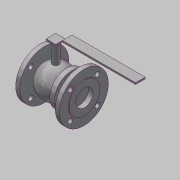
# Autodesk Inventor part: BALL VALVE FLANGED DN65
Saved by Autodesk Inventor 2017 (Build 210142000, 142)
## iProperties
Category: Piping Part
Company: Demarec
Created: 2012-12-20
Part Number: BALL VALVE FLANGED DN65
Material: S235
Document SubType Name: Modeling
Designer: Marc Crauwels
Density: 7.85 g/cm^3
Mass: 658107 g
Surface Area: 21375.3 cm^2
Volume: 83622.3 cm^3
Appearance: Steel
Description: BELVEN BV4
Author: Marc Crauwels
Title: Carbon Steel Globe Valve PN16
Comments: iPart CS GlbVlvPN16
Autodesk Inventor part; units mm, degrees
ref_plane "YZ Plane" through (0, 0, 0) normal (1, 0, 0) x (0, 1, 0)
ref_plane "XZ Plane" through (0, 0, 0) normal (0, 1, 0) x (-1, 0, 0)
sketch "Sketch1" plane through (0, 0, 0) normal (1, 0, 0) x (0, 1, 0)
  line L0 (67, 32.5) -> (83, 32.5)
  line L1 (83, 32.5) -> (83, 92.5)
  line L2 (83, 92.5) -> (67, 92.5)
  line L3 (67, 92.5) -> (67, 32.5)
  line L4 (83, 32.5) -> (85, 32.5)
  line L5 (85, 32.5) -> (85, 58.5)
  line L6 (85, 58.5) -> (83, 58.5)
  line L7 (83, 58.5) -> (83, 32.5)
  line L8 (-85, 0) -> (85, 0) construction
  line L9 (85, 0) -> (67, 0) construction
  line L10 (0, 0) -> (0, 98.124) construction
  line L11 (-85, 0) -> (-67, 0) construction
  line L12 (0, 0) -> (-17.7833, 0)
  dimension "Lenght" = 170
  dimension "DN" = 65
  dimension "FlgDia" = 185
  dimension "FlgThck" = 18
  dimension "GsktFace" = 117
  dimension "Face" = 2
  constraints: 26 end point, 5 point on line, 4 parallel, 3 horizontal, 3 perpendicular, 2 coincident, 2 collinear, 1 midpoint
  measures "Lenght" distance of L8.start L8.end
  measures "DN" diameter of L0 L8
  measures "FlgDia" diameter of L2 L8
  measures "FlgThck" distance between parallel lines of L3 L5
  measures "GsktFace" diameter of L5.end L8
  measures "Face" distance of L5.end L6.end
revolve "Revolution1" add sketch "Sketch1" angle 360 about axis through (0, -85, 0) along (0, 1, 0)
sketch "Sketch5" plane through (0, 83, 0) normal (0, 1, 0) x (1, 0, 0)
  line L0 (0, 0) -> (-51.2652, 51.2652)
  line L1 (0, 0) -> (0, 103.939) construction
  circle A0 centre (-51.2652, 51.2652) radius 9
  point P0 (0, 0)
  dimension "d16" = 72.5
  dimension "d17" = 45
  dimension "d18" = 18
  constraints: 4 end point, 2 coincident, 1 centre point, 1 vertical
  measures "d16" distance of L0.start L0.end
  measures "d17" angle of L1 L0
  measures "d18" diameter of A0
extrude "Extrusion2" cut sketch "Sketch5" against normal through all
pattern_circular "Circular Pattern1" count 4 over 360 about axis through (0, 84, 0) along (0, 1, 0) of "Extrusion2"
sketch "Sketch14" plane through (0, 67, 0) normal (0, -1, 0) x (-1, 0, 0)
  circle A0 centre (0, 0) radius 32.5 projected
  circle A1 centre (0, 0) radius 42.5
  dimension "d54" = 10
  constraints: 1 centre point
  measures "d54" radial gap between concentric circles of A1 A0
pattern_circular "Circular Pattern2" count 2 over 360 about axis through (-10, 0, 0) along (1, 0, 0) of "Revolution1", "Extrusion2", "Circular Pattern1"
extrude "Extrusion5" add sketch "Sketch14" along normal up to surface (134 mm away) contours A0 | A1
sketch "Sketch20" plane through (0, 0, 0) normal (1, 0, 0) x (0, 1, 0)
  line L0 (24, -60.75) -> (24, 60.75)
  arc A0 (24, -60.75) -> (24, 60.75) centre (24, 0) ccw
  line L1 (85, -67.3299) -> (85, 28.8182)
  line L2 (24, 0) -> (36.15, 0)
  line L3 (36.15, 0) -> (36.15, 133)
  line L4 (36.15, 133) -> (24, 133)
  line L5 (24, 133) -> (24, 0)
  line L6 (42.225, 133) -> (5.775, 133)
  line L7 (5.775, 133) -> (5.775, 139.075)
  line L8 (5.775, 139.075) -> (42.225, 139.075)
  line L9 (42.225, 139.075) -> (42.225, 133)
  line L10 (-19.999, 164.849) -> (-297, 164.849)
  line L11 (-297, 164.849) -> (-297, 158.774)
  line L12 (-297, 158.774) -> (-19.999, 158.774)
  line L13 (-19.999, 158.774) -> (-19.999, 164.849)
  line L14 (-19.999, 158.774) -> (5.775, 133)
  line L15 (5.775, 139.075) -> (-19.999, 164.849)
  line L16 (67, -42.5) -> (67, 42.5) projected
  line L17 (-67, 42.5) -> (-67, -42.5) projected
  line L18 (85, -32.5) -> (85, 32.5) projected
  line L19 (85, -58.5) -> (85, 58.5) projected
  point P0 (0, 0)
  point P1 (24, -8.4077)
  point P2 (24, -8.4077)
  point P3 (85, -67.3299)
  point P4 (85, 28.8182)
  dimension "d78" = 121.5
  dimension "oI" = 61
  dimension "oH" = 133
  dimension "d81" = 12.15
  dimension "d85" = 135
  dimension "d86" = 6.075
  dimension "d87" = 6.075
  dimension "oW" = 321
  dimension "d89" = 36.45
  constraints: 30 end point, 7 parallel, 3 horizontal, 3 perpendicular, 2 midpoint, 2 point on circle, 2 vertical, 1 centre point, 1 equal length, 1 point on line, 7 other
  measures "d78" distance of L0.start L0.end
  measures "oH" distance of L4.end L2.start
  measures "d81" distance of L4.end L3.end
  measures "d85" angle of L15 L8
  measures "d86" distance from line of L6.start L3
  measures "d87" distance of L8.end L6.start
  measures "oW" distance between parallel lines of L11 L5
  measures "d89" distance of L7.end L8.end
revolve "Revolution5" add sketch "Sketch20" angle 360 about axis through (0, 24, 133) along (0, 0, -1) contours L0 L2 L3 A0 | L0 A0 L3 L2 | A0 L5 L4 L3
extrude "Extrusion8" add sketch "Sketch20" along normal mid plane 36.45 contours L4 L6 L7 L8 L9 | L14 L13 L15 L7 | L12 L11 L10 L13
ref_plane "Work Plane1" through (0, -36.75, 0) normal (0, -1, 0) x (1, 0, 0)
sketch "Sketch21" plane through (0, -36.75, 0) normal (0, -1, 0) x (1, 0, 0)
  circle A0 centre (0, 0) radius 42.5 projected
  circle A1 centre (0, 0) radius 65
  point P0 (0, 0)
  dimension "d92" = 130
  constraints: 1 centre point, 1 coincident
  measures "d92" diameter of A1
extrude "Extrusion9" add sketch "Sketch21" against normal blind 18
equation "\"d16\" = 0.5 * KDia"
equation "\"KDia\" = 145"
body "Solid1"
